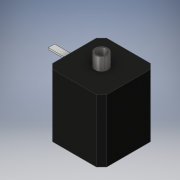
# Autodesk Inventor part: L4118L1804-T6X1 — LINEAR ACTUATOR
Saved by Autodesk Inventor 2018 (Build 220112000, 112)
## iProperties
Created: 2017-12-20
Part Number: L4118L1804-T6X1 — LINEAR ACTUATOR
Material: Generic
Document SubType Name: Modeling
Designer: MISAKA
Density: 1 g/cm^3
Appearance: Black
Author: MISAKA
Autodesk Inventor part; units mm, degrees
ref_plane "YZ Plane" through (0, 0, 0) normal (1, 0, 0) x (0, 1, 0)
ref_plane "XZ Plane" through (0, 0, 0) normal (0, 1, 0) x (-1, 0, 0)
ref_plane "XY Plane" through (0, 0, 0) normal (0, 0, 1) x (1, 0, 0)
sketch "Sketch1" plane through (0, 0, 0) normal (0, 1, 0) x (-1, 0, 0)
  line L0 (-21.15, 21.15) -> (21.15, 21.15)
  line L1 (21.15, 21.15) -> (21.15, -21.15)
  line L2 (21.15, -21.15) -> (-21.15, -21.15)
  line L3 (-21.15, -21.15) -> (-21.15, 21.15)
  line L4 (-21.15, 21.15) -> (21.15, -21.15) construction
  line L5 (21.15, 21.15) -> (-21.15, -21.15) construction
  circle A0 centre (0, 0) radius 3
  circle A1 centre (0, 0) radius 11
  line L6 (15.5, 15.5) -> (-15.5, 15.5)
  line L7 (-15.5, 15.5) -> (-15.5, -15.5)
  line L8 (-15.5, -15.5) -> (15.5, -15.5)
  line L9 (15.5, -15.5) -> (15.5, 15.5)
  line L10 (15.5, 15.5) -> (-15.5, -15.5) construction
  line L11 (-15.5, 15.5) -> (15.5, -15.5) construction
  dimension "d0" = 42.3
  dimension "d10" = 6
  dimension "d11" = 22
  dimension "d18" = 31
  constraints: 24 end point, 4 midpoint, 4 parallel, 3 perpendicular, 2 centre point, 2 coincident, 2 horizontal, 1 point on line
  measures "d0" distance between parallel lines of L2 L0
  measures "d10" diameter of A0
  measures "d11" diameter of A1
  measures "d18" distance of L7.end L8.end
extrude "Extrusion1" add sketch "Sketch1" along normal blind 49 contours L0 L1 L2 L3 | A1 | L9 L8 L7 L6
sketch "Sketch2" plane through (-21.15, 0, -21.15) normal (-1, 0, 0) x (0, 0, 1)
  line L0 (25.6555, 40.0488) -> (16.6445, 40.0488)
  line L1 (16.6445, 40.0488) -> (16.6445, 45.3886)
  line L2 (16.6445, 45.3886) -> (25.6555, 45.3886)
  line L3 (25.6555, 45.3886) -> (25.6555, 40.0488)
  line L4 (25.6555, 40.0488) -> (16.6445, 45.3886) construction
  line L5 (16.6445, 40.0488) -> (25.6555, 45.3886) construction
  line L6 (42.3, 0) -> (0, 0) projected
  point P0 (21.15, 0)
  point P1 (21.15, 42.7187)
  point P2 (21.15, 40.0488)
  point P3 (21.15, 0)
  constraints: 12 end point, 4 midpoint, 2 parallel, 1 horizontal, 1 perpendicular, 1 vertical alignment
extrude "Extrusion2" cut sketch "Sketch2" against normal blind 2
sketch "Sketch3" plane through (-19.15, 0, -21.15) normal (-1, 0, 0) x (0, 0, 1)
  line L0 (25.6555, 40.0488) -> (16.6445, 40.0488) projected
  line L1 (25.6555, 45.3886) -> (25.6555, 40.0488) projected
  line L2 (16.6445, 45.3886) -> (25.6555, 45.3886) projected
  line L3 (16.6445, 40.0488) -> (16.6445, 45.3886) projected
  line L4 (18.676, 42.0802) -> (23.624, 42.0802)
  line L5 (23.624, 42.0802) -> (23.624, 43.3572)
  line L6 (23.624, 43.3572) -> (18.676, 43.3572)
  line L7 (18.676, 43.3572) -> (18.676, 42.0802)
  point P0 (21.15, 0)
  constraints: 8 end point, 3 other
extrude "Extrusion3" add sketch "Sketch3" along normal blind 20 contours L7 L6 L5 L4
chamfer "Chamfer1" distance 4 angle 45 4 edges at (-21.15, 24.5, 21.15) (21.15, 24.5, 21.15) (21.15, 24.5, -21.15) (-21.15, 24.5, -21.15)
extrude "Extrusion4" add sketch "Sketch1" against normal blind 2 contours A1
sketch "Sketch4" plane through (0, 49, 0) normal (0, 1, 0) x (1, 0, 0)
  circle A0 centre (0, 0) radius 5
  circle A1 centre (0, 0) radius 4
  dimension "d14" = 10
  dimension "d15" = 1
  constraints: 2 centre point, 2 coincident
  measures "d14" diameter of A0
  measures "d15" radial gap between concentric circles of A1 A0
extrude "Extrusion5" add sketch "Sketch4" along normal blind 10
hole "Hole1" at (-15.5, 0, -15.5) at (15.5, 0, -15.5) at (15.5, 0, 15.5) at (-15.5, 0, 15.5) direction (0, 1, 0) diameter 2.459 depth 8.8 tip angle 118 thread size "M3x0.5" class "6H" standard "ISO Metric profile"
body "Solid1"
